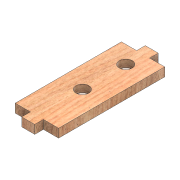
# Autodesk Inventor part: MidjuHaldarar
Saved by Autodesk Inventor 2018 (Build 220112000, 112)
## iProperties
Created: 2020-03-01
Part Number: MidjuHaldarar
Material: Wood (Birch)
Document SubType Name: Modeling
Designer: Spark
Density: 0.55 g/cm^3
Appearance: Birch - Natural Polished
Author: Spark
Autodesk Inventor part; units mm, degrees
ref_plane "YZ Plane" through (0, 0, 0) normal (1, 0, 0) x (0, 1, 0)
ref_plane "XZ Plane" through (0, 0, 0) normal (0, 1, 0) x (-1, 0, 0)
ref_plane "XY Plane" through (0, 0, 0) normal (0, 0, 1) x (1, 0, 0)
sketch "Sketch1" plane through (0, 0, 0) normal (0, 0, 1) x (1, 0, 0)
  line L0 (0, 0) -> (100, 0)
  line L1 (100, 0) -> (100, 285)
  line L2 (100, 285) -> (0, 285)
  line L3 (0, 285) -> (0, 0)
  dimension "d0" = 100
  dimension "d1" = 285
  constraints: 8 end point, 2 parallel, 1 horizontal, 1 perpendicular
  measures "d0" distance of L2.end L1.end
  measures "d1" distance of L0.end L1.end
extrude "Extrusion1" add sketch "Sketch1" along normal blind 20
sketch "Sketch2" plane through (0, 0, 0) normal (0, 0, -1) x (-1, 0, 0)
  circle A0 centre (-50, 125) radius 15
  circle A1 centre (-50, 225) radius 15
  line L0 (0, 285) -> (0, 0) projected
  line L1 (0, 0) -> (-100, 0) projected
  dimension "d5" = 30
  dimension "d6" = 50
  dimension "d7" = 50
  dimension "d9" = 100
  dimension "d13" = 125
  constraints: 2 centre point, 1 equal radius
  measures "d5" diameter of A0
  measures "d6" distance from line of L0 A1.centre
  measures "d7" distance from line of L0 A0.centre
  measures "d9" distance of A1.centre A0.centre
  measures "d13" distance from line of L1 A0.centre
extrude "Extrusion2" cut sketch "Sketch2" against normal up to next
sketch "Sketch3" plane through (0, 0, 20) normal (0, 0, 1) x (1, 0, 0)
  line L0 (0, 0) -> (100, 0) projected
  line L1 (100, 285) -> (0, 285) projected
  line L2 (35, 285) -> (35, 265)
  line L3 (0, 285) -> (0, 0) projected
  line L4 (100, 0) -> (100, 285) projected
  line L5 (35, 265) -> (0, 265)
  line L6 (65, 285) -> (65, 265)
  line L7 (65, 265) -> (100, 265)
  line L8 (35, 0) -> (35, 20)
  line L9 (35, 20) -> (0, 20)
  line L10 (65, 0) -> (65, 20)
  line L11 (100, 20) -> (65, 20)
  dimension "d14" = 30
  dimension "d26" = 35
  dimension "d27" = 20
  dimension "d28" = 20
  constraints: 16 end point, 14 point on line, 4 perpendicular, 1 collinear, 1 horizontal, 1 vertical
  measures "d14" distance between parallel lines of L6 L2
  measures "d26" distance of L2.end L5.end
  measures "d27" distance between parallel lines of L1 L5
  measures "d28" distance between parallel lines of L0 L9
extrude "Extrusion3" cut sketch "Sketch3" against normal up to next contours L3 L9 L8 L0 | L10 L11 L4 L0 | L3 L1 L2 L5 | L7 L6 L1 L4
sketch "Sketch5" plane through (100, 20, 0) normal (1, 0, 0) x (0, 0, -1)
  line L0 (-20, 0) -> (-20, 245) projected
  line L1 (-20, 122.5) -> (-90.7107, 193.2107) construction
  line L2 (-20, 122.5) -> (80, 122.5) construction
  line L3 (-20, 265) -> (0, 265) projected
  point P0 (0, -20)
  dimension "d21" = 100
  dimension "d22" = 135
  dimension "d23" = 142.5
  constraints: 4 end point, 1 equal length, 1 horizontal, 1 midpoint
  measures "d21" distance of L1.start L1.end
  measures "d22" angle of L2 L1
  measures "d23" distance from line of L3 L1.start
fillet "Fillet1" radius 3 2 edges at (65, 125, 0) (65, 225, 0)
body "Solid1"
